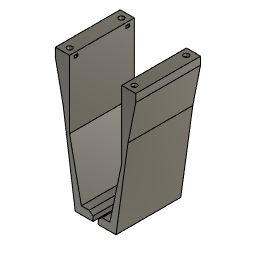
craneproject (Autodesk Fusion 360 archive; units mm, degrees)
design "Claw"
Autodesk Fusion 360 part; units mm, degrees
note: some values were not read from the file. Set by a fixed rule: which face or edge a step refers to.
sketch "Sketch1" plane through (0, 0, 0) normal (0, 0, 1) x (1, 0, 0)
  line L0 (0, 25) -> (25, 25)
  line L1 (25, 25) -> (25, 0)
  line L2 (25, 0) -> (0, 0)
  line L3 (0, 0) -> (0, 25)
  constraint horizontal L0
  constraint vertical L1
  constraint horizontal L2
  constraint vertical L3
extrude "Extrude1" add sketch "Sketch1" along normal blind 40 contours L0 L1 L2 L3 picked at (8.333333, 16.666667) makes body 1
sketch "Sketch2" plane through (0, 25, 0) normal (0, 1, 0) x (-1, 0, 0)
  line L0 (-25, 0) -> (0, 0)
  line L1 (0, 0) -> (0, 40)
  line L2 (0, 40) -> (-25, 40)
  line L3 (-25, 40) -> (-25, 0)
  line L4 (-25, 33) -> (-25, 40)
  line L5 (-20.372796, 0) -> (0, 0)
  line L6 (-25, 33) -> (-20.372796, 0)
  line L7 (-12.5, 40) -> (-12.5, 0)
  line L8 (0, 33) -> (-4.627204, 0)
  line L9 (-12.5, 0) -> (-12.5, 3)
  line L10 (-12.5, 3) -> (-18, 3)
  line L11 (-18, 3) -> (-25, 36.5)
  line L12 (-7, 3) -> (0, 36.5)
  line L13 (-12.5, 3) -> (-7, 3)
  line L14 (-15, 3) -> (-12.5, 1)
  line L15 (-10, 3) -> (-12.5, 1)
  line L16 (-25, 40) -> (-22.555865, 40)
  line L17 (-22.555865, 24.803068) -> (-22.555865, 40)
  line L18 (-2.444135, 24.803068) -> (-2.444135, 40)
  line L19 (-25, 50.000001) -> (-22.555865, 50.000001)
  line L20 (-22.555865, 50.000001) -> (-22.555865, 40)
  line L21 (-22.555865, 40) -> (-25, 40)
  line L22 (-25, 40) -> (-25, 50.000001)
  line L23 (0, 50.000001) -> (-2.444135, 50.000001)
  line L24 (-2.444135, 50.000001) -> (-2.444135, 40)
  line L25 (-2.444135, 40) -> (0, 40)
  line L26 (0, 40) -> (0, 50.000001)
  line L27 (-13.511656, 1.809325) -> (-13.5, 0)
  line L28 (-11.488344, 1.809325) -> (-11.5, 0)
  line L29 (-12.5, 7.498844) -> (-6, 7.498844)
  line L30 (-6, 7.498844) -> (-6, 5)
  line L31 (-6, 5) -> (-12.5, 5)
  line L32 (-12.5, 5) -> (-12.5, 7.498844)
  line L33 (-12.5, 7.498844) -> (-19, 7.498844)
  line L34 (-19, 7.498844) -> (-19, 5)
  line L35 (-19, 5) -> (-12.5, 5)
  point P0 (-25, 0)
  dimension "d3" = 33
  dimension "d4" = 7.98188
  constraint coincident L2.end L3.start
  constraint coincident L0.end L1.start
  constraint coincident L4 P0
  constraint coincident L5 P0
  constraint midpoint L2 L7.start
  constraint perpendicular L2 L7
  constraint symmetric L4.start L7 L8.start
  constraint coincident L7 L9.end
  constraint perpendicular L5 L9
  constraint perpendicular L9 L10
  constraint midpoint L4 L11.end
  constraint symmetric L7 L9.end L10.start
  constraint symmetric L7 L10.end L12.start
  constraint symmetric L7 L11.end L12.end
  constraint coincident L10 L14.start
  constraint coincident L9 L14.end
  constraint symmetric L7 L14.start L15.start
  constraint symmetric L7 L14.end L15.end
  constraint perpendicular L3 L16
  constraint perpendicular L16 L17
  constraint horizontal L19
  constraint vertical L20
  constraint horizontal L21
  constraint vertical L22
  constraint horizontal L23
  constraint vertical L24
  constraint horizontal L25
  constraint vertical L26
  constraint coincident L5 L27.end
  constraint symmetric L7 L27.end L28.end
  constraint horizontal L29
  constraint vertical L30
  constraint horizontal L31
  constraint vertical L32
  constraint symmetric L7 L30.end L34.end
  constraint symmetric L7 L31.end L32.start
  measures "d3" distance of L4.start P0
  measures "d4" angle of L4 L6
extrude "Extrude2" cut sketch "Sketch2" against normal blind 25 contours L0 L3 L6 | L7 L9 L10 L14 | L2 L7 L11 L17 L33 | L7 L9 L13 L15 | L7 L10 L11 L35 | L7 L11 L32 L33 L35 | L0 L1 L5 L8 | L7 L12 L13 L31 | L2 L7 L12 L18 L29 | L7 L12 L29 L31 L32 picked at (-23.457599, 11) picked at (-13.670552, 2.603108) picked at (-15.851955, 24.100637) picked at (-11.329448, 2.603108) picked at (-15.30597, 4.333333) picked at (-16.619323, 6.665896) picked at (-1.542401, 11) picked at (-9.69403, 4.333333) picked at (-9.148045, 24.100637) picked at (-8.380677, 6.665896) bodies 1
extrude "Extrude3" add sketch "Sketch2" against normal blind 25 contours L2 L16 L19 L20 L21 L22 | L2 L23 L24 L25 L26 picked at (-24.185288, 46.666667) picked at (-1.629423, 46.666667) bodies 1
extrude "Extrude4" cut sketch "Sketch2" against normal blind 25 contours L0 L5 L7 L9 L14 L27 | L0 L5 L7 L9 L15 L28 picked at (-13.170552, 0.936442) picked at (-11.829448, 0.936442) bodies 1 makes body 2 at (23.457599, 16.666667, 22)
sketch "Sketch3" plane through (0, 0, 50.000001) normal (0, 0, 1) x (-1, 0, 0)
  line L0 (-2.444135, -25) -> (0, -25)
  line L1 (0, -25) -> (0, 0)
  line L2 (0, 0) -> (-2.444135, 0)
  line L3 (-2.444135, 0) -> (-2.444135, -25)
  line L4 (-12.5, 0) -> (-12.5, -25)
  circle A0 centre (-1.25, -5) radius 1
  line L5 (0, -12.5) -> (-2.730828, -12.5)
  circle A1 centre (-1.25, -20) radius 1
  circle A2 centre (-23.749999, -5) radius 1
  circle A3 centre (-23.749999, -20) radius 1
  dimension "d11" = 2
  constraint vertical L4
  constraint midpoint L1 L5.start
  constraint perpendicular L1 L5
  constraint symmetric A0 L5 A1
  constraint symmetric L4 A0 A2
  constraint symmetric L4 A1 A3
  measures "d11" diameter of A0
extrude "Extrude5" cut sketch "Sketch3" against normal blind 2 contours A0 | A1 | A2 | A3 picked at (-1.324174, -4.675024) picked at (-1.27491, -19.711819) picked at (-23.824173, -4.675024) picked at (-24.246276, -20.159313) bodies 1 2
sketch "Sketch4" plane through (0, 0, 48.000001) normal (0, 0, 1) x (-1, 0, 0)
  circle A0 centre (-23.749999, -20) radius 1
  line L0 (-22.999999, -19.4) -> (-23.499999, -19.4)
  line L1 (-23.499999, -19.4) -> (-23.499999, -20.5)
  line L2 (-23.499999, -20.5) -> (-22.999999, -20.5)
  line L3 (-22.999999, -20.5) -> (-22.999999, -19.4)
  line L4 (-12.5, -19.7) -> (-12.5, -17.5)
  line L5 (-1.5, -19.4) -> (-1.5, -20.5)
  line L6 (-1.5, -20.5) -> (-2, -20.5)
  line L7 (-2, -20.5) -> (-2, -19.4)
  line L8 (-2, -19.4) -> (-1.5, -19.4)
  constraint horizontal L0
  constraint vertical L1
  constraint horizontal L2
  constraint vertical L3
  constraint vertical L4
extrude "Extrude6" add sketch "Sketch4" along normal blind 3 separate body contours L0 L1 L2 L3 | L5 L6 L7 L8 picked at (-23.333333, -19.766666) picked at (-1.833333, -19.766666) makes body 3 at (22.999999, 20.133333, 49.000001) makes body 4 at (1.5, 19.766666, 49.000001)
sketch "Sketch5" plane through (2, 0, 0) normal (1, 0, 0) x (0, 1, 0)
  line L0 (19.4, 48.000001) -> (20.5, 48.000001)
  line L1 (19.4, 48.000001) -> (20.5, 48.000001)
  line L2 (20.5, 48.000001) -> (20.5, 49.199999)
  line L3 (20.5, 49.199999) -> (19.4, 49.199999)
  line L4 (19.4, 49.199999) -> (19.4, 48.000001)
  line L5 (12.5, 51.500001) -> (12.5, 53.500001)
  line L6 (4.500001, 48.000001) -> (4.500001, 49.199999)
  line L7 (4.500001, 49.199999) -> (5.600001, 49.199999)
  line L8 (5.600001, 49.199999) -> (5.600001, 48.000001)
  line L9 (5.600001, 48.000001) -> (4.500001, 48.000001)
  constraint horizontal L1
  constraint vertical L2
  constraint horizontal L3
  constraint vertical L4
  constraint vertical L5
sketch "Sketch6" plane through (22.999999, 0, 0) normal (-1, 0, 0) x (0, -1, 0)
  line L0 (-20.5, 48.000001) -> (-19.4, 48.000001)
  line L1 (-19.4, 48.000001) -> (-19.4, 51.000001)
  line L2 (-19.4, 51.000001) -> (-20.5, 51.000001)
  line L3 (-20.5, 51.000001) -> (-20.5, 48.000001)
  line L4 (-20.5, 48.000001) -> (-19.4, 48.000001)
  line L5 (-19.4, 48.000001) -> (-19.4, 49.199999)
  line L6 (-19.4, 49.199999) -> (-20.5, 49.199999)
  line L7 (-20.5, 49.199999) -> (-20.5, 48.000001)
  line L8 (-12.5, 49.500001) -> (-12.5, 47.000001)
  line L9 (-5.600001, 48.000001) -> (-5.600001, 49.199999)
  line L10 (-5.600001, 49.199999) -> (-4.500001, 49.199999)
  line L11 (-4.500001, 49.199999) -> (-4.500001, 48.000001)
  line L12 (-4.500001, 48.000001) -> (-5.600001, 48.000001)
  constraint horizontal L4
  constraint vertical L5
  constraint horizontal L6
  constraint vertical L7
  constraint vertical L8
extrude "Extrude7" cut sketch "Sketch6" along normal blind 1.5 contours L0 L1 L3 L4 L5 L6 L7 picked at (-20.133333, 48.8) bodies 2
extrude "Extrude8" cut sketch "Sketch6" along normal blind 1.3 contours L9 L10 L11 L12 picked at (-5.233334, 48.8) bodies 2
extrude "Extrude9" cut sketch "Sketch5" along normal blind 1.6 contours L6 L7 L8 L9 picked at (4.866667, 48.8) bodies 1
extrude "Extrude10" cut sketch "Sketch5" along normal blind 1 contours L0 L1 L2 L3 L4 picked at (19.766666, 48.8) bodies 1
extrude "Extrude11" add 2 faces at (23.793532, 1.334265, 50.000001) (1.206468, 1.334265, 50.000001) along direction (0, 0, 1) blind 0.5 on bodies 1 2 bodies 2 1
sketch "Sketch7" plane through (2.444135, 0, 0) normal (1, 0, 0) x (0, 1, 0)
  line L0 (19.4, 49.199999) -> (20.5, 49.199999)
  line L1 (20.5, 49.199999) -> (20.5, 48.000001)
  line L2 (20.5, 48.000001) -> (19.4, 48.000001)
  line L3 (19.4, 48.000001) -> (19.4, 49.199999)
  line L4 (5.600001, 48.000001) -> (4.500001, 48.000001)
  line L5 (4.500001, 48.000001) -> (4.500001, 49.199999)
  line L6 (4.500001, 49.199999) -> (5.600001, 49.199999)
  line L7 (5.600001, 49.199999) -> (5.600001, 48.000001)
  line L8 (25, 24.803068) -> (25, 50.500001)
  line L9 (25, 50.500001) -> (0, 50.500001)
  line L10 (0, 50.500001) -> (0, 24.803068)
  line L11 (0, 24.803068) -> (25, 24.803068)
  line L12 (0, 50.500001) -> (25, 50.500001)
  line L13 (25, 50.500001) -> (25, 47.999979)
  line L14 (25, 47.999979) -> (0, 47.999979)
  line L15 (0, 47.999979) -> (0, 50.500001)
  constraint horizontal L12
  constraint vertical L13
  constraint horizontal L14
  constraint vertical L15
extrude "Extrude12" add sketch "Sketch7" against normal blind 1 contours L0 L1 L3 L5 L6 L7 L8 L9 L10 L12 L13 L14 L15 picked at (1.5, 49.233326) bodies 1
sketch "Sketch8" plane through (0, 0, 0) normal (-1, 0, 0) x (0, -1, 0)
  line L0 (-25, 33) -> (0, 33)
  line L1 (0, 33) -> (0, 50.500001)
  line L2 (0, 50.500001) -> (-25, 50.500001)
  line L3 (-25, 50.500001) -> (-25, 33)
  line L4 (-25, 50.500001) -> (0, 50.500001)
  line L5 (0, 50.500001) -> (0, 47.000001)
  line L6 (0, 47.000001) -> (-25, 47.000001)
  line L7 (-25, 47.000001) -> (-25, 50.500001)
  constraint horizontal L4
  constraint vertical L5
  constraint horizontal L6
  constraint vertical L7
extrude "Extrude13" add sketch "Sketch8" against normal blind 1 contours L1 L2 L3 L4 L5 L6 L7 picked at (-16.666667, 49.333334) bodies 1
extrude "Extrude14" add 1 faces at (0, 8.333333, 38.833334) along direction (-1, 0, 0) blind 3 on bodies 1 bodies 1
extrude "Extrude15" add 3 faces at (25, 16.666667, 35.333333) (25, 16.666667, 43.333334) (25, 16.666667, 50.333334) along direction (1, 0, 0) blind 3 on bodies 2 bodies 2
extrude "Extrude16" add 2 faces at (26.185288, 25, 46.833334) (-0.185288, 25, 44.666667) along direction (0, -1, 0) blind 22 on bodies 1 2 bodies 2 1
sketch "Sketch9" plane through (0, 25, 0) normal (0, 1, 0) x (-1, 0, 0)
  line L0 (-13.5, 0) -> (-13.511656, 1.809325)
  line L1 (-13.511656, 1.809325) -> (-15, 3)
  line L2 (-15, 3) -> (-18, 3)
  line L3 (-18, 3) -> (-22.555865, 24.803068)
  line L4 (-22.555865, 24.803068) -> (-22.555865, 50.500001)
  line L5 (-22.555865, 50.500001) -> (-28, 50.500001)
  line L6 (-28, 50.500001) -> (-28, 33)
  line L7 (-28, 33) -> (-25, 33)
  line L8 (-25, 33) -> (-20.372796, 0)
  line L9 (-20.372796, 0) -> (-13.5, 0)
  line L10 (0, 33) -> (3, 47.500001)
  line L11 (3, 47.500001) -> (3, 33)
  line L12 (3, 33) -> (0, 33)
  line L13 (-25, 33) -> (-28, 48.002591)
  line L14 (-28, 33) -> (-25, 33)
  constraint vertical L11
  constraint perpendicular L11 L12
  constraint coincident L7.end L8.start
  constraint coincident L6.end L7.start
extrude "Extrude17" cut sketch "Sketch9" against normal blind 47 contours L6 L7 L13 L14 | L10 L11 L12 picked at (-27, 38.000864) picked at (2, 37.833334) bodies 1 2
sketch "Sketch10" plane through (0, 0, 50.500001) normal (0, 0, 1) x (-1, 0, 0)
  line L0 (-22.555865, -25) -> (-22.555865, 0)
  line L1 (-22.555865, 0) -> (-28, 0)
  line L2 (-28, 0) -> (-28, -25)
  line L3 (-28, -25) -> (-22.555865, -25)
  circle A0 centre (0, -2.5) radius 1
  line L4 (-12.5, -1.8) -> (-12.5, -2.9)
  line L5 (0, -12.5) -> (1.267351, -12.5)
  circle A1 centre (0, -22.5) radius 1
  circle A2 centre (-24.999999, -22.5) radius 1
  circle A3 centre (-24.999999, -2.5) radius 1
  dimension "d38" = 2
  constraint vertical L4
  constraint horizontal L5
  constraint symmetric A0 L5 A1
  constraint symmetric A0 L4 A3
  constraint symmetric L4 A1 A2
  measures "d38" diameter of A0
extrude "Extrude18" cut sketch "Sketch10" against normal blind 1.5 contours A0 | A1 | A2 | A3 picked at (-0.263802, -2.678514) picked at (-0.080617, -22.217774) picked at (-25.496276, -22.659313) picked at (-25.123437, -2.167599) bodies 1 2
sketch "Sketch11" plane through (0, 0, 49.000001) normal (0, 0, 1) x (-1, 0, 0)
  circle A0 centre (-24.999999, -22.5) radius 1
  line L0 (-24.499999, -21.8) -> (-25.499999, -21.8)
  line L1 (-25.499999, -21.8) -> (-25.499999, -23.199999)
  line L2 (-25.499999, -23.199999) -> (-24.499999, -23.199999)
  line L3 (-24.499999, -23.199999) -> (-24.499999, -21.8)
  line L4 (-12.5, -12.5) -> (-14, -12.5)
  line L5 (-24.499999, -1.800001) -> (-24.499999, -3.200001)
  line L6 (-25.499999, -3.200001) -> (-25.499999, -1.800001)
  line L7 (-25.499999, -1.800001) -> (-24.499999, -1.800001)
  line L8 (-24.499999, -3.200001) -> (-25.499999, -3.200001)
  line L9 (-12.5, -8.7) -> (-12.5, -9.5)
  constraint horizontal L0
  constraint vertical L1
  constraint horizontal L2
  constraint vertical L3
  constraint horizontal L4
  constraint vertical L9
extrude "Extrude19" add sketch "Sketch11" along normal blind 2 separate body contours L0 L1 L2 L3 | L5 L6 L7 L8 picked at (-25.166666, -22.266666) picked at (-25.166666, -2.266668) makes body 5 at (24.499999, 22.733333, 49.666667) makes body 6 at (24.499999, 2.266668, 49.666667)
extrude "Extrude20" cut 1 faces at (0.263802, 2.678514, 49.000001) along direction (0, 0, -1) blind 0.5 on bodies 1 bodies 1
extrude "Extrude21" cut 1 faces at (0.080617, 22.217774, 49.000001) along direction (0, 0, -1) blind 0.5 on bodies 1 bodies 1
extrude "Extrude22" cut 1 faces at (25.496276, 22.659313, 49.000001) along direction (0, 0, -1) blind 0.5 on bodies 2 bodies 2
sketch "Sketch12" plane through (24.499999, 0, 0) normal (-1, 0, 0) x (0, -1, 0)
  line L0 (-23.199999, 49.000001) -> (-21.8, 49.000001)
  line L1 (-21.8, 49.000001) -> (-21.8, 51.000001)
  line L2 (-21.8, 51.000001) -> (-23.199999, 51.000001)
  line L3 (-23.199999, 51.000001) -> (-23.199999, 49.000001)
  line L4 (-23.199999, 49.000001) -> (-21.8, 49.000001)
  line L5 (-21.8, 49.000001) -> (-21.8, 50.000001)
  line L6 (-21.8, 50.000001) -> (-23.199999, 50.000001)
  line L7 (-23.199999, 50.000001) -> (-23.199999, 49.000001)
  line L8 (-3.2, 48.999999) -> (-1.8, 48.999999)
  line L9 (-1.8, 48.999999) -> (-1.8, 49.999999)
  line L10 (-1.8, 49.999999) -> (-3.2, 49.999999)
  line L11 (-3.2, 49.999999) -> (-3.2, 48.999999)
  constraint horizontal L4
  constraint vertical L5
  constraint horizontal L6
  constraint vertical L7
  constraint horizontal L8
  constraint vertical L9
  constraint horizontal L10
  constraint vertical L11
extrude "Extrude23" cut sketch "Sketch12" along normal blind 24 contours L8 L9 L10 L11 picked at (-2.733333, 49.666666) bodies 1 2
sketch "Sketch13" plane through (24.499999, 0, 0) normal (-1, 0, 0) x (0, -1, 0)
  line L0 (-23.199999, 49.000001) -> (-21.8, 49.000001)
  line L1 (-21.8, 49.000001) -> (-21.8, 51.000001)
  line L2 (-21.8, 51.000001) -> (-23.199999, 51.000001)
  line L3 (-23.199999, 51.000001) -> (-23.199999, 49.000001)
  line L4 (-23.199999, 49.000001) -> (-21.8, 49.000001)
  line L5 (-21.8, 49.000001) -> (-21.8, 50.000001)
  line L6 (-21.8, 50.000001) -> (-23.199999, 50.000001)
  line L7 (-23.199999, 50.000001) -> (-23.199999, 49.000001)
  constraint horizontal L4
  constraint vertical L5
  constraint horizontal L6
  constraint vertical L7
extrude "Extrude24" cut sketch "Sketch13" along normal blind 25 contours L0 L1 L3 L4 L5 L6 L7 picked at (-22.733333, 49.666667) bodies 1 2
extrude "Extrude25" add 2 faces at (27.300323, 9.311295, 50.500001) (-2.300323, 9.311295, 50.500001) along direction (0, 0, 1) blind 0.5 on bodies 1 2 bodies 2 1
hidden bodies 3 4 5 6
